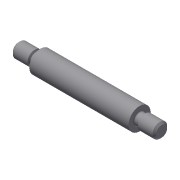
# Autodesk Inventor part: Pin Seized
Saved by Autodesk Inventor 2022 Beta2 (Build 260130000, 130) ContinuousBuild 0
## iProperties
Created: 2006-01-31
Part Number: Pin Seized
Document SubType Name: Modeling
Designer: landrews
Stock Number: Pin Seized
Density: 1 g/cm^3
Material: Generic
Appearance: Default
Author: landrews
Autodesk Inventor part; units mm, degrees
ref_plane "YZ Plane" through (0, 0, 0) normal (1, 0, 0) x (0, 1, 0)
ref_plane "XZ Plane" through (0, 0, 0) normal (0, 1, 0) x (-1, 0, 0)
ref_plane "XY Plane" through (0, 0, 0) normal (0, 0, 1) x (1, 0, 0)
sketch "Sketch1" plane through (0, 0, 0) normal (0, 0, 1) x (1, 0, 0)
  line L0 (-46.8, 0) -> (62.4, 0) projected
  line L1 (0, 7.8) -> (0, -0.6) projected
  line L2 (-39, 0) -> (-39, 4)
  line L3 (-39, 4) -> (-30.0485, 4)
  line L4 (-30.0485, 4) -> (-29.5, 3.05)
  line L5 (-29.5, 3.05) -> (-27, 3.05)
  line L6 (-27, 3.05) -> (-27, 6)
  line L7 (-27, 6) -> (27, 6)
  line L8 (27, 6) -> (27, 3.05)
  line L9 (27, 3.05) -> (29.5, 3.05)
  line L10 (29.5, 3.05) -> (30.0485, 4)
  line L11 (30.0485, 4) -> (39, 4)
  line L12 (39, 4) -> (39, 0)
  line L13 (-39, 0) -> (39, 0)
  dimension "d0" = 4
  dimension "d1" = 60
  dimension "d2" = 12
  dimension "d3" = 78
  dimension "d4" = 3.05
  dimension "d5" = 60
  dimension "d6" = 4
  dimension "d7" = 12
  dimension "d8" = 6
  dimension "d9" = 2.5
  dimension "d10" = 2.5
  dimension "d11" = 3.05
  constraints: 24 end point, 6 parallel, 2 collinear, 2 perpendicular, 2 point on line, 1 other
  measures "d0" distance of L2.start L2.end
  measures "d1" angle of L4 L3
  measures "d2" distance between parallel lines of L6 L2
  measures "d3" distance between parallel lines of L12 L2
  measures "d4" distance between parallel lines of L0 L9
  measures "d5" angle of L11 L10
  measures "d6" distance of L11.end L12.end
  measures "d7" distance between parallel lines of L12 L8
  measures "d8" distance between parallel lines of L13 L7
  measures "d9" distance of L8.end L9.end
  measures "d10" distance of L4.end L5.end
  measures "d11" distance between parallel lines of L13 L5
revolve "Revolution1" add sketch "Sketch1" angle 360 about axis through (-39, 0, 0) along (1, 0, 0)
chamfer "Chamfer1" distance 1 angle 45 2 edges at (39, -4, 0) (-39, -4, 0)
fillet "Fillet1" radius 0.6 2 edges at (-27, -3.05, 0) (27, -3.05, 0)
body "Solid1"
